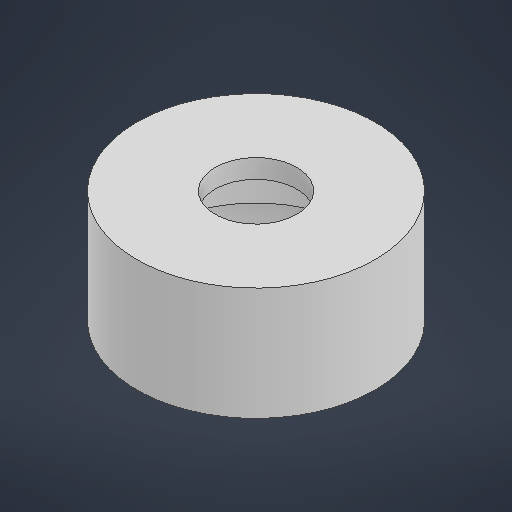
# Autodesk Inventor part: tapa seccion alimentacion
Saved by Autodesk Inventor 2026.1 (Build 301233020, 233B)
## iProperties
Created: 2025-12-03
Part Number: tapa seccion alimentacion
Material: Genérico
Document SubType Name: Modeling
Designer: benja
Density: 1 g/cm^3
Appearance: Valor por defecto
Author: benja
Autodesk Inventor part; units mm, degrees
ref_plane "YZ Plane" through (0, 0, 0) normal (1, 0, 0) x (0, 1, 0)
ref_plane "XZ Plane" through (0, 0, 0) normal (0, 1, 0) x (-1, 0, 0)
ref_plane "XY Plane" through (0, 0, 0) normal (0, 0, 1) x (1, 0, 0)
sketch "Boceto4" plane through (0, 0, 0) normal (0, 1, 0) x (-1, 0, 0)
  circle A0 centre (0, 0) radius 17.05
  circle A1 centre (0, 0) radius 19
  dimension "d10" = 34.1
  dimension "d11" = 38
  constraints: 2 centre point, 2 coincident
  measures "d10" diameter of A0
  measures "d11" diameter of A1
extrude "Extrusión4" add sketch "Boceto4" against normal blind 18
sketch "Boceto5" plane through (0, 0, 0) normal (0, 1, 0) x (1, 0, 0)
  circle A0 centre (0, 0) radius 17.05
  constraints: 1 centre point, 1 coincident
extrude "Extrusión5" add sketch "Boceto5" against normal blind 3
sketch "Boceto6" plane through (0, -3, 0) normal (0, -1, 0) x (1, 0, 0)
  circle A0 centre (0, 0) radius 6.5
  dimension "d16" = 13
  constraints: 1 centre point, 1 coincident
  measures "d16" diameter of A0
extrude "Extrusión6" cut sketch "Boceto6" against normal blind 3
sketch "Boceto7" plane through (0, -3, 0) normal (0, -1, 0) x (1, 0, 0)
  circle A0 centre (0, 0) radius 16
  circle A1 centre (0, 0) radius 6.5 projected
  circle A2 centre (0, 0) radius 16.5
  dimension "d19" = 32
  dimension "d20" = 33
  constraints: 2 centre point, 2 coincident
  measures "d19" diameter of A0
  measures "d20" diameter of A2
extrude "Extrusión7" add sketch "Boceto7" along normal blind 10 contours A2
